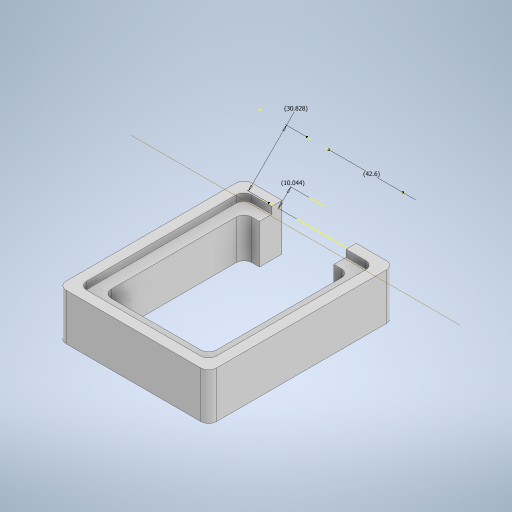
# Autodesk Inventor part: Upper_frame
Saved by Autodesk Inventor 2023 (Build 270158000, 158)
## iProperties
Created: 2023-06-01
Part Number: Upper_frame
Material: Generic
Document SubType Name: Modeling
Designer: Daniil
Density: 1 g/cm^3
Appearance: Default
Author: Daniil
Autodesk Inventor part; units mm, degrees
ref_plane "YZ Plane" through (0, 0, 0) normal (1, 0, 0) x (0, 1, 0)
ref_plane "XZ Plane" through (0, 0, 0) normal (0, 1, 0) x (-1, 0, 0)
ref_plane "XY Plane" through (0, 0, 0) normal (0, 0, 1) x (1, 0, 0)
sketch "Sketch1" plane through (0, 0, 0) normal (0, 1, 0) x (-1, 0, 0)
  line L0 (23.4955, 9.8996) -> (-50.8045, 9.8996)
  line L1 (-50.8045, 9.8996) -> (-50.8045, -84.7004)
  line L2 (-50.8045, -84.7004) -> (23.4955, -84.7004)
  line L3 (23.4955, -84.7004) -> (23.4955, 9.8996)
  line L4 (29.4455, 15.7996) -> (-56.7545, 15.7996)
  line L5 (-56.7545, 15.7996) -> (-56.7545, -90.6004)
  line L6 (-56.7545, -90.6004) -> (29.4455, -90.6004)
  line L7 (29.4455, -90.6004) -> (29.4455, 15.7996)
  line L8 (29.4455, -37.4004) -> (-56.7545, -37.4004) construction
  line L9 (-13.6545, -90.6004) -> (-13.6545, 15.7996) construction
  dimension "d0" = 94.6
  dimension "d1" = 74.3
  dimension "d2" = 106.4
  dimension "d3" = 86.2
  constraints: 20 end point, 4 midpoint, 4 parallel, 2 horizontal, 2 perpendicular, 2 other
  measures "d0" distance between parallel lines of L2 L0
  measures "d1" distance between parallel lines of L1 L3
  measures "d2" distance between parallel lines of L6 L4
  measures "d3" distance between parallel lines of L5 L7
extrude "Extrusion1" add sketch "Sketch1" along normal blind 6
fillet "Fillet1" radius 4.5 4 edges at (-23.4955, 3, 9.8996) (50.8045, 3, 9.8996) (50.8045, 3, -84.7004) (-23.4955, 3, -84.7004)
fillet "Fillet2" radius 4.5 4 edges at (56.7545, 3, 15.7996) (-29.4455, 3, 15.7996) (56.7545, 3, -90.6004) (-29.4455, 3, -90.6004)
sketch "Sketch2" plane through (0, 0, 0) normal (0, -1, 0) x (1, 0, 0)
  line L0 (50.8045, -80.2004) -> (50.8045, 5.3996) projected
  arc A0 (46.3045, -84.7004) -> (50.8045, -80.2004) centre (46.3045, -80.2004) ccw projected
  line L1 (-18.9955, -84.7004) -> (46.3045, -84.7004) projected
  arc A1 (-23.4955, -80.2004) -> (-18.9955, -84.7004) centre (-18.9955, -80.2004) ccw projected
  line L2 (-23.4955, 5.3996) -> (-23.4955, -80.2004) projected
  arc A2 (-18.9955, 9.8996) -> (-23.4955, 5.3996) centre (-18.9955, 5.3996) ccw projected
  line L3 (46.3045, 9.8996) -> (-18.9955, 9.8996) projected
  arc A3 (50.8045, 5.3996) -> (46.3045, 9.8996) centre (46.3045, 5.3996) ccw projected
  line L4 (43.8045, -77.7004) -> (-16.4955, -77.7004)
  line L5 (-16.4955, -77.7004) -> (-16.4955, 2.8996)
  line L6 (-16.4955, 2.8996) -> (43.8045, 2.8996)
  line L7 (43.8045, 2.8996) -> (43.8045, -77.7004)
  line L8 (13.6545, -84.7004) -> (13.6545, 9.8996) construction
  line L9 (46.3045, 9.8996) -> (-18.9955, 9.8996) construction
  line L10 (50.8045, -80.2004) -> (50.8045, 5.3996) construction
  line L11 (50.8045, -37.4004) -> (-23.4955, -37.4004) construction
  line L12 (56.7545, 11.2996) -> (56.7545, -86.1004) construction
  point P0 (0, 0)
  dimension "d8" = 5.95
  dimension "d9" = 7
  dimension "d10" = 7
  constraints: 12 end point, 4 midpoint, 2 parallel, 1 horizontal, 1 perpendicular, 2 other
  measures "d8" distance between parallel lines of L0 L12
  measures "d9" distance between parallel lines of L7 L0
  measures "d10" distance between parallel lines of L1 L4
extrude "Extrusion2" add sketch "Sketch2" along normal blind 6
fillet "Fillet3" radius 4.5 4 edges at (43.8045, -3, -77.7004) (43.8045, -3, 2.8996) (-16.4955, -3, 2.8996) (-16.4955, -3, -77.7004)
sketch "Sketch3" plane through (0, 0, 0) normal (0, 1, 0) x (1, 0, 0)
  arc A0 (46.3045, -9.8996) -> (50.8045, -5.3996) centre (46.3045, -5.3996) ccw projected
  line L0 (50.8045, 80.2004) -> (50.8045, -5.3996) projected
  arc A1 (50.8045, 80.2004) -> (46.3045, 84.7004) centre (46.3045, 80.2004) ccw projected
  line L1 (-18.9955, 84.7004) -> (46.3045, 84.7004) projected
  arc A2 (-18.9955, 84.7004) -> (-23.4955, 80.2004) centre (-18.9955, 80.2004) ccw projected
  line L2 (-23.4955, -5.3996) -> (-23.4955, 80.2004) projected
  arc A3 (-23.4955, -5.3996) -> (-18.9955, -9.8996) centre (-18.9955, -5.3996) ccw projected
  line L3 (46.3045, -9.8996) -> (-18.9955, -9.8996) projected
  arc A4 (43.8045, 73.2004) -> (39.3045, 77.7004) centre (39.3045, 73.2004) ccw projected
  line L4 (43.8045, 1.6004) -> (43.8045, 73.2004) projected
  arc A5 (39.3045, -2.8996) -> (43.8045, 1.6004) centre (39.3045, 1.6004) ccw projected
  line L5 (-11.9955, -2.8996) -> (39.3045, -2.8996) projected
  arc A6 (-16.4955, 1.6004) -> (-11.9955, -2.8996) centre (-11.9955, 1.6004) ccw projected
  line L6 (-16.4955, 73.2004) -> (-16.4955, 1.6004) projected
  arc A7 (-11.9955, 77.7004) -> (-16.4955, 73.2004) centre (-11.9955, 73.2004) ccw projected
  line L7 (39.3045, 77.7004) -> (-11.9955, 77.7004) projected
  point P0 (0, 0)
extrude "Extrusion3" add sketch "Sketch3" along normal blind 2
ref_plane "Work Plane1" through (-23.4955, 6, -84.7004) normal (0, 0.7071068, -0.7071068) x (1, 0, 0)
sketch "Sketch5" plane through (-23.4955, 6, -84.7004) normal (0, 0.7071068, -0.7071068) x (1, 0, 0)
  line L0 (4.5, 0) -> (69.8, 0) projected
  line L1 (37.15, 0) -> (37.15, -42.3796) construction
  circle A0 centre (37.15, 1.34) radius 1.34 construction
  line L2 (37.15, 1.34) -> (37.15, -18.66) construction
  line L3 (38.49, 1.34) -> (38.49, -18.66)
  line L4 (35.81, -18.66) -> (35.81, 1.34)
  arc A1 (38.49, 1.34) -> (35.81, 1.34) centre (37.15, 1.34) ccw
  arc A2 (35.81, -18.66) -> (38.49, -18.66) centre (37.15, -18.66) ccw
  point P0 (23.4955, -55.6496)
  point P1 (37.15, -8.66)
  dimension "d20" = 2.68
  dimension "d19" = 90
  dimension "d21" = 20
  dimension "d22" = 2.68
  constraints: 10 end point, 4 point on circle, 4 tangent, 2 centre point, 2 midpoint, 1 horizontal, 1 parallel, 1 point on line, 1 vertical, 1 vertical alignment, 2 other
  measures "d19" angle of L0 L1
  measures "d21" distance of L2.start L2.end
  measures "d22" distance between parallel lines of L4 L3
extrude "Extrusion5" cut sketch "Sketch5" along normal mid plane 51.82
sketch "Sketch6" plane through (-23.4955, 6, -84.7004) normal (0, 0.7071068, -0.7071068) x (1, 0, 0)
  arc A0 (38.49, 1.34) -> (35.81, 1.34) centre (37.15, 1.34) ccw projected
  line L0 (38.49, 0) -> (38.49, 1.34) projected
  arc A1 (38.49, 1.34) -> (35.81, 1.34) centre (37.15, 1.34) ccw projected
  line L1 (35.81, 1.34) -> (35.81, 0) projected
  line L2 (4.5, 0) -> (35.81, 0) projected
  line L3 (4.5, 2.8284) -> (4.5, 0) projected
  line L4 (4.5, 2.8284) -> (69.8, 2.8284) projected
  line L5 (69.8, 0) -> (69.8, 2.8284) projected
  line L6 (38.49, 0) -> (69.8, 0) projected
  line L7 (75.75, 8.4146) -> (-1.45, 8.4146) projected
  line L8 (74.9473, 2.68) -> (-18.0058, 2.68) construction
  line L9 (0, -55.225) -> (0, 5.3033) construction
  line L10 (90.8097, 9.1284) -> (-67.1811, 9.1284) construction
  line L11 (37.15, 2.68) -> (37.15, 37.6448) construction
  line L12 (58.45, 9.1284) -> (15.85, 9.1284)
  line L13 (15.85, 9.1284) -> (15.85, 13.1284)
  line L14 (15.85, 13.1284) -> (58.45, 13.1284)
  line L15 (58.45, 13.1284) -> (58.45, 9.1284)
  point P0 (23.4955, -55.6496)
  dimension "d25" = 6.3
  dimension "d26" = 42.6
  dimension "d27" = 4
  constraints: 14 end point, 3 perpendicular, 2 horizontal, 2 parallel, 2 point on line, 1 point on circle, 1 tangent, 1 other
  measures "d25" distance between parallel lines of L10 L4
  measures "d26" distance between parallel lines of L13 L15
  measures "d27" distance between parallel lines of L14 L10
extrude "Extrusion6" add sketch "Sketch6" along normal blind 35 contours L12 L13 L14 L15
sketch "Sketch7" plane through (-23.4955, 30.7487, -109.4492) normal (0, 0.7071068, -0.7071068) x (-1, 0, 0)
  line L0 (-15.85, -13.1284) -> (-15.85, -9.1284) projected
  line L1 (-58.45, -9.1284) -> (-58.45, -13.1284) projected
  point P0 (-23.4955, 55.6496)
  point P1 (-15.85, -11.1284)
  point P2 (-58.45, -11.1284)
  dimension "d30" = 42.6
  constraints: 2 midpoint
  measures "d30" distance of point (-15.85, -11.128) point (-58.45, -11.128)
sketch "Sketch8" plane through (34.9545, -3.2832, -93.9836) normal (1, 0, 0) x (0, 0.7071068, -0.7071068)
  line L0 (-0.0707, 4.7139) -> (-3.2527, 7.8958) projected
  line L1 (0.9899, 12.1385) -> (4.1719, 8.9565) projected
  line L2 (0, 0) -> (35, 0) projected
  line L3 (-0.0707, 4.7139) -> (-14.2134, -9.4288) construction
  line L4 (0, 4) -> (35, 4) projected
  line L5 (0, 4) -> (0, 0) projected
  line L6 (4.1719, 8.9565) -> (-4.7846, 0)
  line L7 (-4.7846, 0) -> (0, 0)
  line L8 (0, 0) -> (0, 4) projected
  line L9 (0, 0) -> (0, 4)
  line L10 (4.1719, 8.9565) -> (4.1719, 4)
  line L11 (0, 4) -> (35, 4) projected
  line L12 (4.1719, 4) -> (0, 4)
  line L13 (-0.0707, 4.7139) -> (4.1719, 8.9565) projected
  point P0 (-64.1349, 68.778)
  point P1 (4.1719, 4)
  constraints: 12 end point, 3 point on line, 2 perpendicular, 1 collinear, 1 horizontal, 1 vertical
extrude "Extrusion7" add sketch "Sketch8" against normal blind 42.6
sketch "Sketch9" plane through (34.9545, -6.6664, -90.6004) normal (1, 0, 0) x (0, 0, -1)
  line L0 (0, 6.6664) -> (0, 0) projected
  line L1 (0, 0) -> (28.1319, 28.1319) projected
  line L2 (0, 0) -> (0, 6.6664) projected
  line L3 (0, 0) -> (0, -20)
  line L4 (0, -20) -> (5, -20)
  line L5 (5, -20) -> (5, 5)
  line L6 (0, 0) -> (28.1319, 28.1319) projected
  line L7 (5, 5) -> (0, 0)
  point P0 (-90.6004, 6.6664)
  point P1 (5, 5)
  dimension "d33" = 5
  dimension "d34" = 20
  constraints: 8 end point, 2 perpendicular, 2 point on line, 1 collinear
  measures "d33" distance between parallel lines of L5 L3
  measures "d34" distance from line of L4 L0.end
extrude "Extrusion8" add sketch "Sketch9" against normal blind 42.6
sketch "Sketch10" plane through (-7.6455, 24.294, -115.9039) normal (0, 0.7071068, 0.7071068) x (1, 0, 0)
  line L0 (0, -30.8281) -> (42.6, -30.8281) projected
  line L1 (42.6, -30.8281) -> (42.6, 0) projected
  line L2 (0, 0) -> (42.6, 0) projected
  line L3 (0, -30.8281) -> (0, 0) projected
  line L4 (42.6, -30.8281) -> (0, -30.8281) projected
  line L5 (0, -30.8281) -> (5, -30.8281)
  line L6 (5, -30.8281) -> (5, 0)
  line L7 (5, 0) -> (0, 0)
  line L8 (0, 0) -> (0, -30.8281)
  line L9 (42.6, 0) -> (0, 0) projected
  line L10 (37.6, 0) -> (42.6, 0)
  line L11 (42.6, 0) -> (42.6, -30.8281)
  line L12 (42.6, -30.8281) -> (37.6, -30.8281)
  line L13 (37.6, -30.8281) -> (37.6, 0)
  point P0 (7.6455, -99.1349)
  point P1 (37.6, 0)
  point P2 (37.6, -30.8281)
  dimension "d37" = 5
  dimension "d38" = 5
  constraints: 16 end point, 4 parallel, 2 horizontal, 2 perpendicular, 2 point on line
  measures "d37" distance between parallel lines of L3 L6
  measures "d38" distance between parallel lines of L1 L13
extrude "Extrusion9" add sketch "Sketch10" along normal blind 19 contours L3 L2 L6 L0 | L13 L2 L1 L0
sketch "Sketch11" plane through (-7.6455, 37.729, -102.4689) normal (0, 0.7071068, 0.7071068) x (1, 0, 0)
  line L0 (0, -30.8281) -> (5, -30.8281) projected
  line L1 (5, 0) -> (0, 0) projected
  point P0 (7.6455, -99.1349)
  point P1 (2.5, 0)
  point P2 (2.5, -30.8281)
  dimension "d41" = 30.8281
  constraints: 2 midpoint
  measures "d41" distance of point (2.5, 0) point (2.5, -30.828)
sketch "Sketch12" plane through (-2.6455, 2.4952, -94.1052) normal (1, 0, 0) x (0, -0.7071068, -0.7071068)
  line L0 (0, 30.8281) -> (0, 0) projected
  line L1 (0, 30.8281) -> (-19, 30.8281) projected
  line L2 (-19, 0) -> (-19, 30.8281) projected
  line L3 (-4.9565, 0) -> (-19, 0) projected
  line L4 (0, 0) -> (-4.9565, 0) projected
  line L5 (-19, 30.8281) -> (-15, 30.8281)
  line L6 (-15, 30.8281) -> (-15, 0)
  line L7 (-15, 0) -> (-19, 0)
  line L8 (-19, 0) -> (-19, 30.8281)
  point P0 (-64.778, -68.3068)
  dimension "d42" = 15
  constraints: 8 end point, 2 parallel, 1 horizontal, 1 perpendicular, 1 point on line
  measures "d42" distance between parallel lines of L0 L6
extrude "Extrusion10" add sketch "Sketch12" along normal blind 8.5 contours L6 L3 L2 L1
sketch "Sketch13" plane through (29.9545, 2.4952, -94.1052) normal (-1, 0, 0) x (0, 0.7071068, 0.7071068)
  line L0 (0, 0) -> (0, 30.8281) projected
  line L1 (4.9565, 0) -> (0, 0) projected
  line L2 (4.9565, 0) -> (19, 0) projected
  line L3 (19, 30.8281) -> (19, 0) projected
  line L4 (0, 30.8281) -> (19, 30.8281) projected
  line L5 (19, 30.8281) -> (7.45, 30.8281)
  line L6 (7.45, 30.8281) -> (7.45, 0)
  line L7 (7.45, 0) -> (19, 0)
  line L8 (19, 0) -> (19, 30.8281)
  point P0 (64.778, -68.3068)
  point P1 (7.45, 30.8281)
  dimension "d45" = 7.45
  constraints: 8 end point, 2 parallel, 1 horizontal, 1 perpendicular, 1 point on line
  measures "d45" distance between parallel lines of L6 L0
extrude "Extrusion11" add sketch "Sketch13" along normal blind 8.5 contours L4 L3 L2 L6
sketch "Sketch14" plane through (34.9545, -26.6664, -90.6004) normal (1, 0, 0) x (0, 0, -1)
  line L0 (5, 25) -> (28.1319, 48.1319) projected
  line L1 (28.1319, 48.1319) -> (11.8685, 64.3954) projected
  line L2 (-9.9303, 42.5967) -> (11.8685, 64.3954) projected
  line L3 (0, 32.6664) -> (-9.9303, 42.5967) projected
  line L4 (0, 26.6664) -> (0, 32.6664) projected
  line L5 (0, 26.6664) -> (0, 0) projected
  line L6 (0, 0) -> (5, 0) projected
  line L7 (5, 0) -> (5, 25) projected
  line L8 (0, 32.6664) -> (3.5048, 29.1616) construction
  line L9 (-9.9303, 42.5967) -> (11.8685, 64.3954) construction
  line L10 (-7.1018, 39.7682) -> (14.6969, 61.567) construction
  line L11 (0, 32.6664) -> (-1.7632, 34.4296) projected
  line L12 (0, 52.5269) -> (0, 32.6664)
  line L13 (-1.7632, 34.4296) -> (-9.9303, 42.5967) projected
  line L14 (0, 32.6664) -> (-9.9303, 42.5967)
  line L15 (-9.9303, 42.5967) -> (0, 52.5269)
  point P0 (-90.6004, 26.6664)
  point P1 (11.8685, 64.3954)
  point P2 (0, 52.5269)
  constraints: 6 end point, 2 collinear, 1 coincident, 1 perpendicular, 1 point on line
extrude "Extrusion12" cut sketch "Sketch14" against normal blind 100 contours L12 L3 L2
sketch "Sketch15" plane through (-23.4955, 30.7487, -109.4492) normal (0, 0.7071068, -0.7071068) x (-1, 0, 0)
  line L0 (-58.45, -13.1284) -> (-15.85, -13.1284) projected
  line L1 (-15.85, -13.1284) -> (-15.85, 9.8716) projected
  line L2 (-15.85, 9.8716) -> (-29.35, 9.8716) projected
  line L3 (-29.35, 5.8716) -> (-29.35, 9.8716) projected
  line L4 (-20.85, 5.8716) -> (-29.35, 5.8716) projected
  line L5 (-20.85, -9.1284) -> (-20.85, 5.8716) projected
  line L6 (-20.85, -9.1284) -> (-53.45, -9.1284) projected
  line L7 (-53.45, -9.1284) -> (-53.45, -1.6784) projected
  line L8 (-53.45, -1.6784) -> (-44.95, -1.6784) projected
  line L9 (-44.95, 9.8716) -> (-44.95, -1.6784) projected
  line L10 (-58.45, 9.8716) -> (-44.95, 9.8716) projected
  line L11 (-58.45, -13.1284) -> (-58.45, 9.8716) projected
  line L12 (-58.45, 9.8716) -> (-44.95, 9.8716)
  line L13 (-44.95, 9.8716) -> (-44.95, 2.3216)
  line L14 (-44.95, 2.3216) -> (-58.45, 2.3216)
  line L15 (-58.45, 2.3216) -> (-58.45, 9.8716)
  point P0 (-23.4955, 55.6496)
  point P1 (-51.7, 2.3216)
  point P2 (-58.45, 2.3216)
  dimension "d52" = 4
  constraints: 8 end point, 2 parallel, 1 horizontal, 1 midpoint, 1 perpendicular, 1 point on line
  measures "d52" distance from line of L8 point (-51.7, 2.322)
extrude "Extrusion13" cut sketch "Sketch15" against normal blind 100 contours L11 L10 L9 L14
sketch "Sketch16" plane through (-2.6455, 24.294, -115.9039) normal (0, 0.7071068, 0.7071068) x (1, 0, 0)
  line L0 (32.6, -30.8281) -> (0, -30.8281) projected
  line L1 (8.5, -20.7846) -> (0, -20.7846) projected
  point P0 (2.6455, -99.1349)
  dimension "d55" = 10.0435
  measures "d55" distance between parallel lines of L1 L0
sketch "Sketch17" plane through (-2.6455, 6, -90.6004) normal (1, 0, 0) x (0, 0, -1)
  line L0 (0, 14.2037) -> (0, 0) projected
  line L1 (3.5048, -3.5048) -> (0, 0) projected
  line L2 (25.3035, 18.294) -> (3.5048, -3.5048) projected
  line L3 (25.3035, 18.294) -> (14.6969, 28.9006) projected
  line L4 (14.6969, 28.9006) -> (0, 14.2037) projected
  line L5 (5.6261, -1.3835) -> (3.5048, -3.5048)
  line L6 (3.5048, -3.5048) -> (0, 0)
  line L7 (0, 0) -> (2.1213, 2.1213)
  line L8 (2.1213, 2.1213) -> (5.6261, -1.3835)
  point P0 (-90.6004, -6)
  dimension "d56" = 3
  constraints: 8 end point, 2 parallel, 1 perpendicular, 1 point on line
  measures "d56" distance between parallel lines of L1 L8
extrude "Extrusion14" add sketch "Sketch17" along normal blind 34.75 contours L7 L8 L2 L1
sketch "Sketch18" plane through (0, -6, 0) normal (0, -1, 0) x (1, 0, 0)
  line L0 (-18.9955, -84.7004) -> (46.3045, -84.7004) projected
  line L1 (39.3045, -77.7004) -> (-11.9955, -77.7004) projected
  line L2 (-7.6455, -95.6004) -> (-7.6455, -90.6004) projected
  line L3 (34.9545, -90.6004) -> (34.9545, -95.6004) projected
  line L4 (-18.9955, -84.7004) -> (46.3045, -84.7004) projected
  line L5 (-7.6455, -84.7004) -> (34.9545, -84.7004)
  line L6 (34.9545, -84.7004) -> (34.9545, -77.7004)
  line L7 (34.9545, -77.7004) -> (-7.6455, -77.7004)
  line L8 (-7.6455, -77.7004) -> (-7.6455, -84.7004)
  point P0 (0, 0)
  constraints: 8 end point, 2 collinear, 2 parallel, 2 point on line, 1 horizontal, 1 perpendicular
extrude "Extrusion15" add sketch "Sketch18" along normal blind 20
fillet "Fillet5" radius 5 2 edges at (5.8545, 36.3148, -103.8831) (21.4545, 30.9761, -109.2218)
sketch "Sketch19" plane through (0, 6, 0) normal (0, 1, 0) x (1, 0, 0)
  line L0 (14.9945, 86.5955) -> (14.9945, 84.7004) projected
  line L1 (14.9945, 84.7004) -> (46.3045, 84.7004) projected
  arc A0 (50.8045, 80.2004) -> (46.3045, 84.7004) centre (46.3045, 80.2004) ccw projected
  line L2 (50.8045, 80.2004) -> (50.8045, -5.3996) projected
  arc A1 (46.3045, -9.8996) -> (50.8045, -5.3996) centre (46.3045, -5.3996) ccw projected
  line L3 (46.3045, -9.8996) -> (-18.9955, -9.8996) projected
  arc A2 (-23.4955, -5.3996) -> (-18.9955, -9.8996) centre (-18.9955, -5.3996) ccw projected
  line L4 (-23.4955, -5.3996) -> (-23.4955, 80.2004) projected
  arc A3 (-18.9955, 84.7004) -> (-23.4955, 80.2004) centre (-18.9955, 80.2004) ccw projected
  line L5 (-18.9955, 84.7004) -> (12.3145, 84.7004) projected
  line L6 (12.3145, 84.7004) -> (12.3145, 86.5955) projected
  ellipse E0 centre (13.6545, 86.5955) end of major axis (13.6545, 88.4905) minor radius 1.34 (14.9945, 86.5955) -> (12.3145, 86.5955) ccw projected
  arc A4 (-24.9455, 90.6004) -> (-29.4455, 86.1004) centre (-24.9455, 86.1004) ccw projected
  line L7 (-29.4455, 86.1004) -> (-29.4455, -11.2996) projected
  arc A5 (-29.4455, -11.2996) -> (-24.9455, -15.7996) centre (-24.9455, -11.2996) ccw projected
  line L8 (-24.9455, -15.7996) -> (52.2545, -15.7996) projected
  arc A6 (52.2545, -15.7996) -> (56.7545, -11.2996) centre (52.2545, -11.2996) ccw projected
  line L9 (56.7545, -11.2996) -> (56.7545, 86.1004) projected
  arc A7 (56.7545, 86.1004) -> (52.2545, 90.6004) centre (52.2545, 86.1004) ccw projected
  line L10 (52.2545, 90.6004) -> (34.9545, 90.6004) projected
  line L11 (34.9545, 90.6004) -> (29.9545, 90.6004) projected
  line L12 (29.9545, 90.6004) -> (-2.6455, 90.6004) projected
  line L13 (-2.6455, 90.6004) -> (-7.6455, 90.6004) projected
  line L14 (-7.6455, 90.6004) -> (-24.9455, 90.6004) projected
  point P0 (0, 0)
  constraints: 1 other
extrude "Extrusion16" add sketch "Sketch19" along normal blind 5
sketch "Sketch20" plane through (0, 2, 0) normal (0, 1, 0) x (1, 0, 0)
  line L0 (14.9945, 82.5955) -> (14.9945, 77.7004) projected
  line L1 (14.9945, 77.7004) -> (39.3045, 77.7004) projected
  arc A0 (43.8045, 73.2004) -> (39.3045, 77.7004) centre (39.3045, 73.2004) ccw projected
  line L2 (43.8045, 73.2004) -> (43.8045, 1.6004) projected
  arc A1 (39.3045, -2.8996) -> (43.8045, 1.6004) centre (39.3045, 1.6004) ccw projected
  line L3 (39.3045, -2.8996) -> (-11.9955, -2.8996) projected
  arc A2 (-16.4955, 1.6004) -> (-11.9955, -2.8996) centre (-11.9955, 1.6004) ccw projected
  line L4 (-16.4955, 1.6004) -> (-16.4955, 73.2004) projected
  arc A3 (-11.9955, 77.7004) -> (-16.4955, 73.2004) centre (-11.9955, 73.2004) ccw projected
  line L5 (-11.9955, 77.7004) -> (12.3145, 77.7004) projected
  line L6 (12.3145, 77.7004) -> (12.3145, 82.5955) projected
  ellipse E0 centre (13.6545, 82.5955) end of major axis (13.6545, 84.4905) minor radius 1.34 (14.9945, 82.5955) -> (12.3145, 82.5955) ccw projected
  line L7 (46.3045, -9.8996) -> (-18.9955, -9.8996) projected
  arc A4 (46.3045, -9.8996) -> (50.8045, -5.3996) centre (46.3045, -5.3996) ccw projected
  line L8 (50.8045, 80.2004) -> (50.8045, -5.3996) projected
  arc A5 (50.8045, 80.2004) -> (46.3045, 84.7004) centre (46.3045, 80.2004) ccw projected
  line L9 (-18.9955, 84.7004) -> (46.3045, 84.7004) projected
  arc A6 (-18.9955, 84.7004) -> (-23.4955, 80.2004) centre (-18.9955, 80.2004) ccw projected
  line L10 (-23.4955, -5.3996) -> (-23.4955, 80.2004) projected
  arc A7 (-23.4955, -5.3996) -> (-18.9955, -9.8996) centre (-18.9955, -5.3996) ccw projected
  point P0 (0, 0)
  constraints: 1 other
extrude "Extrusion17" add sketch "Sketch20" along normal blind 5
sketch "Sketch21" plane through (0, 11, 0) normal (0, 1, 0) x (1, 0, 0)
  line L0 (-7.6455, 118.7324) -> (-7.6455, 102.4689) projected
  line L1 (34.9545, 118.7324) -> (34.9545, 107.8076) projected
  line L2 (34.9545, 118.7324) -> (-7.6455, 118.7324) projected
  line L3 (-11.9955, 77.7004) -> (12.3145, 77.7004) projected
  line L4 (14.9945, 77.7004) -> (39.3045, 77.7004) projected
  line L5 (34.9545, 77.7004) -> (-7.6455, 77.7004) projected
  line L6 (-7.6455, 118.7324) -> (34.9545, 118.7324)
  line L7 (34.9545, 118.7324) -> (34.9545, 77.7004)
  line L8 (34.9545, 77.7004) -> (-7.6455, 77.7004)
  line L9 (-7.6455, 77.7004) -> (-7.6455, 118.7324)
  point P0 (0, 0)
  constraints: 8 end point, 2 parallel, 1 horizontal, 1 perpendicular
extrude "Extrusion18" cut sketch "Sketch21" along normal mid plane 100
sketch "Sketch22" plane through (0, 0, 0) normal (0, -1, 0) x (1, 0, 0)
  line L0 (87.9396, -104.4246) -> (-53.0165, -104.4246)
  line L1 (-53.0165, -104.4246) -> (-53.0165, 23.665)
  line L2 (-53.0165, 23.665) -> (87.9396, 23.665)
  line L3 (87.9396, 23.665) -> (87.9396, -104.4246)
  point P0 (0, 0)
  constraints: 8 end point, 2 parallel, 1 horizontal, 1 perpendicular
extrude "Extrusion19" cut sketch "Sketch22" along normal blind 100
sketch "Sketch23" plane through (0, 0, 0) normal (0, -1, 0) x (1, 0, 0)
  line L0 (34.9545, -77.7004) -> (34.9545, -90.6004) projected
  line L1 (52.2545, -90.6004) -> (34.9545, -90.6004) projected
  arc A0 (52.2545, -90.6004) -> (56.7545, -86.1004) centre (52.2545, -86.1004) ccw projected
  line L2 (56.7545, 11.2996) -> (56.7545, -86.1004) projected
  arc A1 (56.7545, 11.2996) -> (52.2545, 15.7996) centre (52.2545, 11.2996) ccw projected
  line L3 (-24.9455, 15.7996) -> (52.2545, 15.7996) projected
  arc A2 (-24.9455, 15.7996) -> (-29.4455, 11.2996) centre (-24.9455, 11.2996) ccw projected
  line L4 (-29.4455, -86.1004) -> (-29.4455, 11.2996) projected
  arc A3 (-29.4455, -86.1004) -> (-24.9455, -90.6004) centre (-24.9455, -86.1004) ccw projected
  line L5 (-7.6455, -90.6004) -> (-24.9455, -90.6004) projected
  line L6 (-7.6455, -77.7004) -> (-7.6455, -90.6004) projected
  line L7 (-11.9955, -77.7004) -> (-7.6455, -77.7004) projected
  arc A4 (-16.4955, -73.2004) -> (-11.9955, -77.7004) centre (-11.9955, -73.2004) ccw projected
  line L8 (-16.4955, -1.6004) -> (-16.4955, -73.2004) projected
  arc A5 (-11.9955, 2.8996) -> (-16.4955, -1.6004) centre (-11.9955, -1.6004) ccw projected
  line L9 (39.3045, 2.8996) -> (-11.9955, 2.8996) projected
  arc A6 (43.8045, -1.6004) -> (39.3045, 2.8996) centre (39.3045, -1.6004) ccw projected
  line L10 (43.8045, -73.2004) -> (43.8045, -1.6004) projected
  arc A7 (39.3045, -77.7004) -> (43.8045, -73.2004) centre (39.3045, -73.2004) ccw projected
  line L11 (34.9545, -77.7004) -> (39.3045, -77.7004) projected
  point P0 (0, 0)
extrude "Extrusion20" add sketch "Sketch23" along normal blind 5.6
sketch "Sketch24" plane through (0, -5.6, 0) normal (0, -1, 0) x (1, 0, 0)
  point P0 (0, 0)
sketch "Sketch25" plane through (0, -5.6, 0) normal (0, -1, 0) x (1, 0, 0)
  line L0 (34.9545, -77.7004) -> (34.9545, -90.6004) projected
  line L1 (34.9545, -90.6004) -> (52.2545, -90.6004) projected
  arc A0 (52.2545, -90.6004) -> (56.7545, -86.1004) centre (52.2545, -86.1004) ccw projected
  line L2 (56.7545, -86.1004) -> (56.7545, 11.2996) projected
  arc A1 (56.7545, 11.2996) -> (52.2545, 15.7996) centre (52.2545, 11.2996) ccw projected
  line L3 (52.2545, 15.7996) -> (-24.9455, 15.7996) projected
  arc A2 (-24.9455, 15.7996) -> (-29.4455, 11.2996) centre (-24.9455, 11.2996) ccw projected
  line L4 (-29.4455, 11.2996) -> (-29.4455, -86.1004) projected
  arc A3 (-29.4455, -86.1004) -> (-24.9455, -90.6004) centre (-24.9455, -86.1004) ccw projected
  line L5 (-24.9455, -90.6004) -> (-7.6455, -90.6004) projected
  line L6 (-7.6455, -90.6004) -> (-7.6455, -77.7004) projected
  line L7 (-7.6455, -77.7004) -> (-11.9955, -77.7004) projected
  arc A4 (-16.4955, -73.2004) -> (-11.9955, -77.7004) centre (-11.9955, -73.2004) ccw projected
  line L8 (-16.4955, -73.2004) -> (-16.4955, -1.6004) projected
  arc A5 (-11.9955, 2.8996) -> (-16.4955, -1.6004) centre (-11.9955, -1.6004) ccw projected
  line L9 (-11.9955, 2.8996) -> (39.3045, 2.8996) projected
  arc A6 (43.8045, -1.6004) -> (39.3045, 2.8996) centre (39.3045, -1.6004) ccw projected
  line L10 (43.8045, -1.6004) -> (43.8045, -73.2004) projected
  arc A7 (39.3045, -77.7004) -> (43.8045, -73.2004) centre (39.3045, -73.2004) ccw projected
  line L11 (39.3045, -77.7004) -> (34.9545, -77.7004) projected
  point P0 (0, 0)
extrude "Extrusion21" add sketch "Sketch25" along normal blind 10
body "Solid1"
